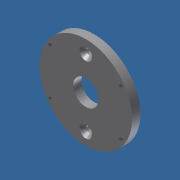
# Autodesk Inventor part: Dewalt Drill Drive CIMmotor Adaptor
Saved by Autodesk Inventor 2012 (Build 160160000, 160)
## iProperties
Created: 2012-07-04
Part Number: Dewalt Drill Drive CIMmotor Adaptor
Material: Default
Document SubType Name: Modeling
Designer: Bruce
Density: 1 g/cm^3
Author: Bruce
Autodesk Inventor part; units mm, degrees
ref_plane "YZ Plane" through (0, 0, 0) normal (1, 0, 0) x (0, 1, 0)
ref_plane "XZ Plane" through (0, 0, 0) normal (0, 1, 0) x (-1, 0, 0)
ref_plane "XY Plane" through (0, 0, 0) normal (0, 0, 1) x (1, 0, 0)
sketch "Sketch1" plane through (0, 0, 0) normal (0, 0, 1) x (1, 0, 0)
  circle A0 centre (0, 0) radius 34.925
  circle A1 centre (0, 0) radius 9.525
  point P0 (0, 25.4)
  point P1 (0, -25.4)
  point P2 (-26.797, -17.4625)
  point P3 (-26.797, 17.4625)
  point P4 (26.797, 17.4625)
  point P5 (26.797, -17.4625)
  dimension "d0" = 69.85
  dimension "d1" = 19.05
  dimension "d2" = 25.4
  dimension "d3" = 25.4
  dimension "d4" = 26.797
  dimension "d5" = 17.4625
  dimension "d6" = 17.4625
  dimension "d7" = 26.797
  constraints: 4 vertical alignment, 2 centre point, 2 coincident, 2 horizontal alignment
  measures "d0" diameter of A0
  measures "d1" diameter of A1
  measures "d2" distance of point (0, 0) point (0, 25.4)
  measures "d3" distance of point (0, -25.4) point (0, 0)
  measures "d4" horizontal distance of point (-26.797, -17.463) point (0, 0)
  measures "d5" vertical distance of point (-26.797, -17.463) point (0, 0)
  measures "d6" vertical distance of point (0, 0) point (-26.797, 17.463)
  measures "d7" horizontal distance of point (26.797, -17.463) point (0, 0)
extrude "Extrusion1" add sketch "Sketch1" against normal blind 6.35
hole "Hole1" at (-26.797, -17.4625, 0) at (-26.797, 17.4625, 0) at (26.797, 17.4625, 0) at (26.797, -17.4625, 0) direction (0, 0, -1) diameter 2.6416 end through all thread size "6-32 UNC" class "2B" standard "ANSI Unified Screw Threads"
hole "Hole2" at (0, 25.4, 0) at (0, -25.4, 0) direction (0, 0, -1) diameter 4.826 end through all countersink diameter 9.525 countersink angle 82
body "Solid1"
